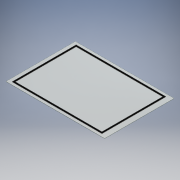
# Autodesk Inventor part: magnifier
Saved by Autodesk Inventor 2016 (Build 200138000, 138)
## iProperties
Created: 2023-11-17
Part Number: magnifier
Material: Glass
Document SubType Name: Modeling
Designer: Zizi
Mass: 70.3181 g
Surface Area: 927.704 cm^2
Volume: 32.256 cm^3
Density: 2.18 g/cm^3
Appearance: Clear
Author: Zizi
Autodesk Inventor part; units mm, degrees
ref_plane "YZ Plane" through (0, 0, 0) normal (1, 0, 0) x (0, 1, 0)
ref_plane "XZ Plane" through (0, 0, 0) normal (0, 1, 0) x (-1, 0, 0)
ref_plane "XY Plane" through (0, 0, 0) normal (0, 0, 1) x (1, 0, 0)
sketch "Magnifier_Sketch" plane through (0, 0, 0) normal (0, 0, 1) x (1, 0, 0)
  line L0 (0, 0) -> (256, 0)
  line L1 (256, 0) -> (256, 180)
  line L2 (256, 180) -> (0, 180)
  line L3 (0, 180) -> (0, 0)
  dimension "d0" = 180
  dimension "d1" = 256
  constraints: 8 end point, 2 parallel, 1 horizontal, 1 perpendicular
  measures "d0" distance of L2.end L0.start
  measures "d1" distance of L0.start L0.end
extrude "Magnifier_Extrusion" add sketch "Magnifier_Sketch" along normal blind 0.7
sketch "FrontLine_Sketch" plane through (0, 0, 0.7) normal (0, 0, 1) x (1, 0, 0)
  line L0 (242, 173) -> (9, 173)
  line L1 (9, 173) -> (9, 7)
  line L2 (9, 7) -> (242, 7)
  line L3 (242, 7) -> (242, 173)
  line L4 (0, 180) -> (0, 0) projected
  line L5 (256, 180) -> (0, 180) projected
  line L6 (256, 0) -> (256, 180) projected
  line L7 (0, 0) -> (256, 0) projected
  line L8 (13, 11) -> (13, 169)
  line L9 (13, 169) -> (238, 169)
  line L10 (238, 169) -> (238, 11)
  line L11 (238, 11) -> (13, 11)
  dimension "d4" = 9
  dimension "d5" = 7
  dimension "d6" = 14
  dimension "d7" = 7
  dimension "d9" = 4
  constraints: 16 end point, 4 parallel, 2 perpendicular, 1 horizontal, 3 other
  measures "d4" distance between parallel lines of L4 L1
  measures "d5" distance between parallel lines of L5 L0
  measures "d6" distance between parallel lines of L6 L3
  measures "d7" distance between parallel lines of L7 L2
  measures "d9" distance between parallel lines of L1 L8
extrude "FrontLine_Extrusion" add sketch "FrontLine_Sketch" along normal blind 0.3 separate body contours L3 L2 L1 L0
sketch "BackLine_Sketch" plane through (0, 0, 0) normal (0, 0, -1) x (-1, 0, 0)
  line L0 (-13, 169) -> (-238, 169) projected
  line L1 (-238, 169) -> (-238, 11) projected
  line L2 (-238, 11) -> (-13, 11) projected
  line L3 (-13, 11) -> (-13, 169) projected
  line L4 (-242, 173) -> (-9, 173) projected
  line L5 (-9, 173) -> (-9, 7) projected
  line L6 (-9, 7) -> (-242, 7) projected
  line L7 (-242, 7) -> (-242, 173) projected
  point P0 (0, 0)
extrude "Extrusion3" add sketch "BackLine_Sketch" along normal blind 0.3 separate body
equation "\"d0\" = magnifier_h"
equation "\"d1\" = magnifier_w"
equation "\"d2\" = magnifier_d"
equation "\"d4\" = magnifier_l"
equation "\"d5\" = magnifier_t"
equation "\"d6\" = magnifier_r"
equation "\"d7\" = magnifier_b"
equation "\"d9\" = magnifier_line_w"
equation "\"d10\" = magnifier_line_d"
equation "\"d12\" = magnifier_line_d"
equation "\"magnifier_w\" = 256"
equation "\"magnifier_h\" = 180"
equation "\"magnifier_d\" = 0.7"
equation "\"magnifier_l\" = 9"
equation "\"magnifier_t\" = 7"
equation "\"magnifier_r\" = 14"
equation "\"magnifier_b\" = 7"
equation "\"magnifier_line_w\" = 4"
equation "\"magnifier_line_d\" = 0.3"
